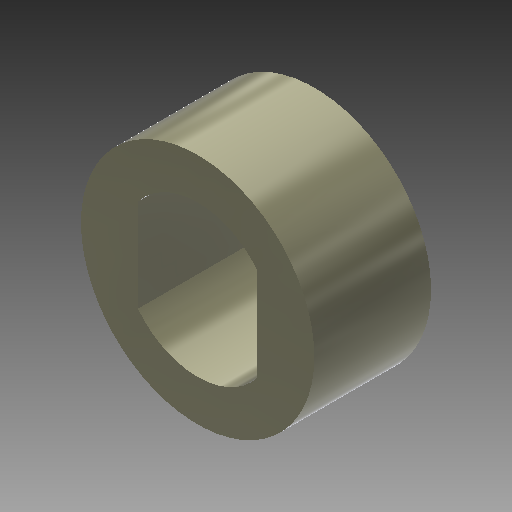
# Autodesk Inventor part: 308-05
Saved by Autodesk Inventor 2019 (Build 230136000, 136)
## iProperties
Company: Autodesk Inc.
Created: 2012-01-25
Part Number: 308-05
Material: Polypropylene
Document SubType Name: Modeling
Designer: Autodesk Inc.
Mass: 0.432336 g
Surface Area: 5.53628 cm^2
Volume: 0.480907 cm^3
Density: 0.899 g/cm^3
Appearance: Smooth - Ash
Author: Inventor
Autodesk Inventor part; units mm, degrees
ref_plane "YZ Plane" through (0, 0, 0) normal (1, 0, 0) x (0, 1, 0)
ref_plane "XZ Plane" through (0, 0, 0) normal (0, 1, 0) x (-1, 0, 0)
ref_plane "XY Plane" through (0, 0, 0) normal (0, 0, 1) x (1, 0, 0)
sketch "Sketch1" plane through (0, 0, 0) normal (0, 0, 1) x (1, 0, 0)
  circle A0 centre (0, 0) radius 6.25
  line L0 (-3.2, 2.4824) -> (-3.2, -2.4824)
  line L1 (3.2, 2.4824) -> (3.2, -2.4824)
  arc A1 (3.2, 2.4824) -> (-3.2, 2.4824) centre (0, 0) ccw
  arc A2 (-3.2, -2.4824) -> (3.2, -2.4824) centre (0, 0) ccw
  dimension "d0" = 12.5
  dimension "d2" = 6.4
  dimension "d3" = 4.05
  constraints: 4 end point, 4 point on circle, 3 centre point, 2 coincident, 2 parallel, 1 concentric, 1 vertical
  measures "d0" diameter of A0
  measures "d2" distance between parallel lines of L1 L0
  measures "d3" radius of A2
extrude "Extrusion1" add sketch "Sketch1" along normal blind 6.25
body "Solid1"
